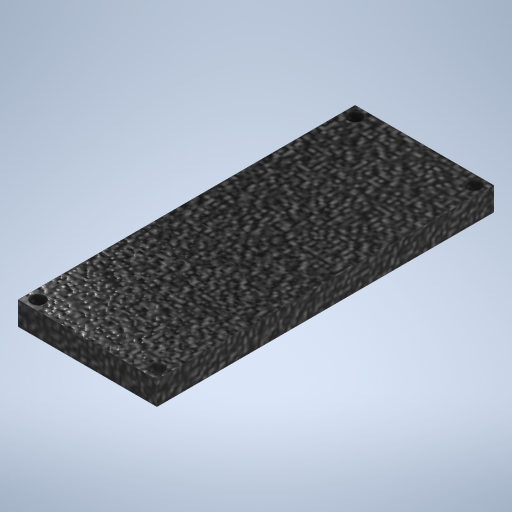
# Autodesk Inventor part: arduino nano screw ports
Saved by Autodesk Inventor 2023 (Build 270158000, 158)
## iProperties
Created: 2023-03-17
Part Number: arduino nano screw ports
Material: Generic
Document SubType Name: Modeling
Designer: user
Density: 1 g/cm^3
Appearance: Black Cast
Author: user
Autodesk Inventor part; units mm, degrees
ref_plane "YZ Plane" through (0, 0, 0) normal (1, 0, 0) x (0, 1, 0)
ref_plane "XZ Plane" through (0, 0, 0) normal (0, 1, 0) x (-1, 0, 0)
ref_plane "XY Plane" through (0, 0, 0) normal (0, 0, 1) x (1, 0, 0)
sketch "Sketch1" plane through (0, 0, 0) normal (0, 1, 0) x (-1, 0, 0)
  line L0 (8.89, 21.59) -> (-8.89, 21.59)
  line L1 (-8.89, 21.59) -> (-8.89, -21.59)
  line L2 (-8.89, -21.59) -> (8.89, -21.59)
  line L3 (8.89, -21.59) -> (8.89, 21.59)
  circle A0 centre (7.62, 20.32) radius 0.889
  circle A1 centre (-7.62, 20.32) radius 0.889
  line L4 (8.89, 0) -> (-8.89, 0) construction
  circle A2 centre (7.62, -20.32) radius 0.889
  circle A3 centre (-7.62, -20.32) radius 0.889
  point P0 (0, 0)
  dimension "d0" = 17.78
  dimension "d1" = 43.18
  dimension "d2" = 21.59
  dimension "d3" = 8.89
  dimension "d4" = 15.24
  dimension "d5" = 7.62
  dimension "d6" = 1.778
  dimension "d7" = 1.778
  dimension "d8" = 1.27
  dimension "d9" = 1.27
  dimension "d10" = 1.27
  dimension "d11" = 40.64
  dimension "d12" = 13.462
  dimension "d15" = 15.24
  constraints: 10 end point, 4 centre point, 2 midpoint, 2 parallel, 2 symmetric about line, 1 horizontal, 1 perpendicular, 2 other
  measures "d0" distance of L2.end L1.end
  measures "d1" distance of L1.end L0.end
  measures "d2" distance from line of point (0, 0) L0
  measures "d3" distance from line of point (0, 0) L3
  measures "d4" distance of A1.centre A0.centre
  measures "d5" horizontal distance of A0.centre point (0, 0)
  measures "d6" diameter of A0
  measures "d7" diameter of A1
  measures "d8" distance from line of L3 A0.centre
  measures "d9" distance from line of L0 A0.centre
  measures "d10" distance from line of L1 A1.centre
  measures "d11" distance of A0.centre A2.centre
  measures "d15" distance of A2.centre A3.centre
extrude "Extrusion1" add sketch "Sketch1" along normal blind 3
equation "\"d2\" = 0.5 * d1"
equation "\"d3\" = 0.5 * d0"
equation "\"d5\" = 0.5 * d4"
equation "\"d9\" = d8"
body "Solid1"
